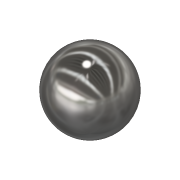
# Autodesk Inventor part: V2_ball_bearing_three_point
Saved by Autodesk Inventor 2019 (Build 230136000, 136)
## iProperties
Created: 2018-07-28
Part Number: V2_ball_bearing_three_point
Material: Generic
Document SubType Name: Modeling
Designer: richp
Density: 1 g/cm^3
Appearance: Default
Author: richp
Autodesk Inventor part; units mm, degrees
ref_plane "YZ Plane" through (0, 0, 0) normal (1, 0, 0) x (0, 1, 0)
ref_plane "XZ Plane" through (0, 0, 0) normal (0, 1, 0) x (-1, 0, 0)
ref_plane "XY Plane" through (0, 0, 0) normal (0, 0, 1) x (1, 0, 0)
sketch "Sketch1" plane through (0, 0, 0) normal (0, 0, 1) x (1, 0, 0)
  circle A0 centre (0, 0) radius 1.1906
  line L0 (-1.6669, 0) -> (1.6669, 0) projected
  line L1 (-1.1906, 0) -> (1.1906, 0)
  dimension "d0" = 2.3813
  constraints: 2 end point, 2 point on circle, 2 point on line, 1 centre point, 1 coincident
  measures "d0" diameter of A0
revolve "Revolution1" add sketch "Sketch1" angle 360 about axis through (-10, 0, 0) along (1, 0, 0) picked at (0.2971, 0.2632) contours L0 A0
equation "\"d0\" = bb_diameter"
equation "\"bb_diameter\" = 2.38125"
body "Solid1"
